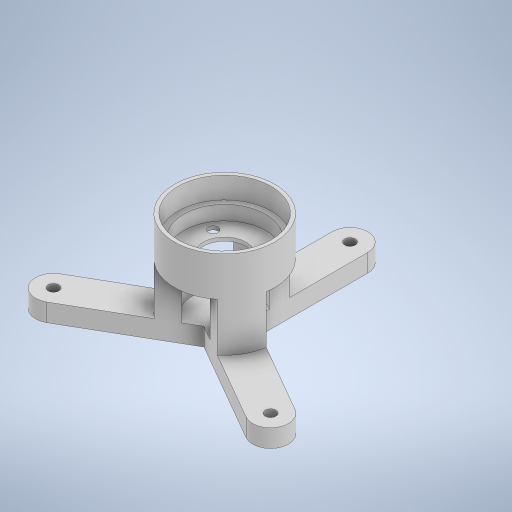
# Autodesk Inventor part: Base
Saved by Autodesk Inventor 2023 (Build 270158000, 158)
## iProperties
Created: 2022-12-10
Part Number: Base
Material: Generic
Document SubType Name: Modeling
Designer: Krzysztof
Density: 1 g/cm^3
Appearance: Default
Author: Krzysztof
## iProperties of the stored document Base_3DPrint.ipt
Created: 2022-12-19
Part Number: Base_3DPrint
Material: Generic
Document SubType Name: Modeling
Designer: Krzysztof
Density: 1 g/cm^3
Appearance: Default
Author: Krzysztof
Autodesk Inventor part; units mm, degrees
ref_plane "YZ Plane" through (0, 0, 0) normal (1, 0, 0) x (0, 1, 0)
ref_plane "XZ Plane" through (0, 0, 0) normal (0, 1, 0) x (-1, 0, 0)
ref_plane "XY Plane" through (0, 0, 0) normal (0, 0, 1) x (1, 0, 0)
sketch "Sketch1" plane through (0, 0, 0) normal (0, 1, 0) x (-1, 0, 0)
  line L0 (0, 0) -> (0, -70) construction
  line L1 (-10, 0) -> (-10, -70)
  line L2 (10, -70) -> (10, 0)
  arc A0 (10, 0) -> (-10, 0) centre (0, 0) ccw
  arc A1 (-10, -70) -> (10, -70) centre (0, -70) ccw
  line L3 (0, 0) -> (60.6218, 35) construction
  line L4 (5, -8.6603) -> (65.6218, 26.3397)
  line L5 (55.6218, 43.6603) -> (-5, 8.6603)
  arc A2 (-5, 8.6603) -> (5, -8.6603) centre (0, 0) ccw
  arc A3 (65.6218, 26.3397) -> (55.6218, 43.6603) centre (60.6218, 35) ccw
  line L6 (0, 0) -> (-60.6218, 35) construction
  line L7 (5, 8.6603) -> (-55.6218, 43.6603)
  line L8 (-65.6218, 26.3397) -> (-5, -8.6603)
  arc A4 (-5, -8.6603) -> (5, 8.6603) centre (0, 0) ccw
  arc A5 (-55.6218, 43.6603) -> (-65.6218, 26.3397) centre (-60.6218, 35) ccw
  circle A6 centre (0, -70) radius 3
  circle A7 centre (60.6218, 35) radius 3
  circle A8 centre (-60.6218, 35) radius 3
  point P0 (0, -35)
  point P1 (30.3109, 17.5)
  point P2 (-30.3109, 17.5)
  point P3 (10, -5.7735)
  point P4 (0, 11.547)
  point P5 (-10, -5.7735)
  dimension "d0" = 20
  dimension "d1" = 70
  dimension "d4" = 360
  dimension "d64" = 6
  dimension "d67" = 360
  constraints: 24 end point, 12 point on circle, 9 centre point, 4 tangent, 3 coincident, 1 midpoint, 1 parallel, 1 vertical, 42 other
  measures "d0" distance between parallel lines of L2 L1
  measures "d1" distance of L0.start L0.end
  measures "d64" diameter of A6
extrude "Extrusion1" add sketch "Sketch1" along normal blind 10
sketch "Sketch2" plane through (0, 10, 0) normal (0, 1, 0) x (1, 0, 0)
  arc A0 (10, 26.1534) -> (-10, 26.1534) centre (0, 0) ccw
  arc A1 (10, 14.9666) -> (-10, 14.9666) centre (0, 0) ccw
  line L0 (-10, 70) -> (-10, 5.7735) projected
  line L1 (-10, 14.9666) -> (-10, 26.1534)
  line L2 (10, 26.1534) -> (10, 14.9666)
  line L3 (10, 5.7735) -> (10, 70) projected
  arc A2 (-27.6495, -4.4164) -> (-17.6495, -21.737) centre (0, 0) ccw
  arc A3 (-17.9615, 1.1769) -> (-7.9615, -16.1436) centre (0, 0) ccw
  line L4 (-7.9615, -16.1436) -> (-17.6495, -21.737)
  line L5 (-27.6495, -4.4164) -> (-17.9615, 1.1769)
  arc A4 (17.6495, -21.737) -> (27.6495, -4.4164) centre (0, 0) ccw
  arc A5 (7.9615, -16.1436) -> (17.9615, 1.1769) centre (0, 0) ccw
  line L6 (17.9615, 1.1769) -> (27.6495, -4.4164)
  line L7 (17.6495, -21.737) -> (7.9615, -16.1436)
  dimension "d38" = 18
  dimension "d39" = 28
  dimension "d42" = 360
  constraints: 12 end point, 12 point on circle, 6 centre point, 4 coincident, 4 point on line, 31 other
  measures "d38" radius of A1
  measures "d39" radius of A0
extrude "Extrusion2" add sketch "Sketch2" along normal blind 27
sketch "Sketch3" plane through (0, 37, 0) normal (0, 1, 0) x (1, 0, 0)
  circle A0 centre (0, 0) radius 12
  circle A1 centre (0, 0) radius 28
  circle A2 centre (0, 0) radius 17.5 construction
  circle A3 centre (0, -17.5) radius 2.75
  line L0 (0, 0) -> (0, -33.6866) construction
  circle A4 centre (15.1554, 8.75) radius 2.75
  circle A5 centre (-15.1554, 8.75) radius 2.75
  dimension "d50" = 35
  dimension "d46" = 56
  dimension "d47" = 24
  dimension "d51" = 5.5
  dimension "d54" = 360
  constraints: 5 centre point, 3 coincident, 2 end point, 1 point on line, 1 vertical, 1 vertical alignment, 9 other
  measures "d46" diameter of A1
  measures "d47" diameter of A0
  measures "d51" diameter of A3
extrude "Extrusion3" add sketch "Sketch3" along normal blind 2
sketch "Sketch4" plane through (0, 39, 0) normal (0, 1, 0) x (1, 0, 0)
  circle A0 centre (0, 0) radius 23
  circle A1 centre (0, 0) radius 28
  dimension "d56" = 46
  dimension "d57" = 56
  constraints: 2 centre point, 2 coincident
  measures "d56" diameter of A0
  measures "d57" diameter of A1
extrude "Extrusion4" add sketch "Sketch4" along normal blind 8
sketch "Sketch5" plane through (0, 47, 0) normal (0, 1, 0) x (1, 0, 0)
  circle A0 centre (0, 0) radius 28
  circle A1 centre (0, 0) radius 26
  dimension "d60" = 56
  dimension "d61" = 52
  constraints: 2 centre point, 2 coincident
  measures "d60" diameter of A0
  measures "d61" diameter of A1
extrude "Extrusion5" add sketch "Sketch5" along normal blind 12
body "Solid1"
